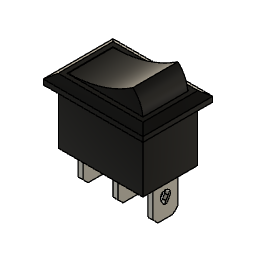
power_switch (Autodesk Fusion 360 design; units mm, degrees)
Autodesk Fusion 360 part; units mm, degrees
sketch "Main body" plane through (0, 0, 0) normal (0, 0, 1) x (1, 0, 0)
  line L0 (0, 0) -> (17, 0)
  line L1 (17, 0) -> (17, 11)
  line L2 (17, 11) -> (0, 11)
  line L3 (0, 11) -> (0, 0)
  dimension "d1" = 17
  dimension "d2" = 11
  constraint horizontal L0
  constraint vertical L1
  constraint horizontal L2
  constraint vertical L3
  constraint coincident L0.start L3.end
  measures "d1" distance of L0.start L0.end
  measures "d2" distance of L0.end L1.end
extrude "Extrude1" add sketch "Main body" along normal blind 11 makes body 1
sketch "Top Plate" plane through (0, 0, 11) normal (0, 0, 1) x (-1, 0, 0)
  line L0 (0, -11) -> (0, 0)
  line L1 (0, 0) -> (-17, 0)
  line L2 (-17, 0) -> (-17, -11)
  line L3 (-17, -11) -> (0, -11)
  line L4 (1.5, -12.5) -> (-18.5, -12.5)
  line L5 (-18.5, -12.5) -> (-18.5, 1.5)
  line L6 (-18.5, 1.5) -> (1.5, 1.5)
  line L7 (1.5, 1.5) -> (1.5, -12.5)
  dimension "d5" = 20
  dimension "d6" = 1.5
  dimension "d7" = 1.5
  dimension "d8" = 14
  dimension "d9" = 1.5
  dimension "d10" = 1.5
  constraint horizontal L4
  constraint vertical L5
  constraint horizontal L6
  constraint vertical L7
  measures "d5" distance of L5.end L6.end
  measures "d6" distance of L0 L7
  measures "d7" distance of L2 L5
  measures "d8" distance of L4.end L5.end
  measures "d9" distance of L3 L4
  measures "d10" distance of L1 L6
extrude "Extrude2" add sketch "Top Plate" along normal blind 2 contours L0 L1 L2 L3 | L4 L5 L6 L7 bodies 1
chamfer "Chamfer1" distance 1.5 distance2 1 1 edges at (8.5, -1.5, 13) measured on face at (11.8333, 7.8333, 13) on bodies 1
chamfer "Chamfer1" distance 1.5 distance2 1 3 edges at (18.5, 5.5, 13) (8.5, 12.5, 13) (-1.5, 5.5, 13) measured on face at (11.8333, 7.8333, 13) measured on face at (11.8333, 7.8333, 13) measured on face at (11.8333, 7.8333, 13) on bodies 1
sketch "Switch" plane through (0, 0, 13) normal (0, 0, 1) x (-1, 0, 0)
  line L0 (-17, -11) -> (0, -11)
  line L1 (0, -11) -> (0, 0)
  line L2 (0, 0) -> (-17, 0)
  line L3 (-17, 0) -> (-17, -11)
  line L4 (-1, -10) -> (-16, -10)
  line L5 (-16, -10) -> (-16, -1)
  line L6 (-16, -1) -> (-1, -1)
  line L7 (-1, -1) -> (-1, -10)
  line L8 (-0.9, -10.1) -> (-16.1, -10.1)
  line L9 (-16.1, -10.1) -> (-16.1, -0.9)
  line L10 (-16.1, -0.9) -> (-0.9, -0.9)
  line L11 (-0.9, -0.9) -> (-0.9, -10.1)
  line L12 (-16, -10) -> (-14, -10)
  line L13 (-14, -10) -> (-14, -1)
  line L14 (-14, -1) -> (-16, -1)
  line L15 (-16, -1) -> (-16, -10)
  dimension "d17" = 1
  dimension "d18" = 1
  dimension "d19" = 1
  dimension "d20" = 1
  dimension "d21" = 0.1
  dimension "d22" = 0.1
  dimension "d23" = 0.1
  dimension "d24" = 0.1
  dimension "d29" = 2
  constraint horizontal L4
  constraint vertical L5
  constraint horizontal L6
  constraint vertical L7
  constraint horizontal L8
  constraint vertical L9
  constraint horizontal L10
  constraint vertical L11
  constraint horizontal L12
  constraint vertical L13
  constraint horizontal L14
  constraint vertical L15
  constraint coincident L6 L13.end
  measures "d17" distance of L0 L4
  measures "d18" distance of L2 L6
  measures "d19" distance of L1 L7
  measures "d20" distance of L3 L5
  measures "d21" distance of L4 L8
  measures "d22" distance of L6 L10
  measures "d23" distance of L7 L11
  measures "d24" distance of L5 L9
  measures "d29" distance of L5 L13
extrude "Extrude3" cut sketch "Switch" against normal blind 1 contours L8 L9 L10 L11 bodies 1
extrude "Extrude4" add sketch "Switch" along normal blind 4 contours L4 L5 L6 L12 L13 L14 L15 bodies 1
fillet "Fillet1" radius 6.25 1 edges at (16, 5.5, 17) on bodies 1
fillet "Fillet2" radius 23.5 1 edges at (14, 5.5, 13) on bodies 1
sketch "Pins" plane through (0, 0, 0) normal (0, 0, -1) x (1, 0, 0)
  line L0 (0, 0) -> (0, -11)
  line L1 (0, -11) -> (17, -11)
  line L2 (17, -11) -> (17, 0)
  line L3 (17, 0) -> (0, 0)
  line L4 (1, -8) -> (2, -8)
  line L5 (2, -8) -> (2, -3)
  line L6 (2, -3) -> (1, -3)
  line L7 (1, -3) -> (1, -8)
  line L8 (8, -8) -> (9, -8)
  line L9 (9, -8) -> (9, -3)
  line L10 (9, -3) -> (8, -3)
  line L11 (8, -3) -> (8, -8)
  line L12 (15, -8) -> (16, -8)
  line L13 (16, -8) -> (16, -3)
  line L14 (16, -3) -> (15, -3)
  line L15 (15, -3) -> (15, -8)
  dimension "d34" = 5
  dimension "d37" = 1
  dimension "d38" = 1
  dimension "d39" = 1
  dimension "d40" = 1
  dimension "d41" = 1
  dimension "d42" = 6
  dimension "d43" = 6
  dimension "d44" = 3
  dimension "d45" = 3
  constraint horizontal L4
  constraint vertical L5
  constraint horizontal L6
  constraint vertical L7
  constraint horizontal L8
  constraint vertical L9
  constraint horizontal L10
  constraint vertical L11
  constraint horizontal L12
  constraint vertical L13
  constraint horizontal L14
  constraint vertical L15
  constraint collinear L6 L10
  constraint collinear L10 L14
  constraint collinear L4 L8
  constraint collinear L8 L12
  measures "d34" distance of L4.start L6.end
  measures "d37" distance of L8.start L8.end
  measures "d38" distance of L4.start L4.end
  measures "d39" distance of L12.start L12.end
  measures "d40" distance of L2 L13
  measures "d41" distance of L0 L7
  measures "d42" distance of L5 L11
  measures "d43" distance of L9 L15
  measures "d44" distance of L3 L6
  measures "d45" distance of L1 L4
extrude "Extrude5" add sketch "Pins" along normal blind 7 separate body contours L4 L5 L6 L7 | L8 L9 L10 L11 | L12 L13 L14 L15 makes body 2 at (1, 4.6667, -2.3333) makes body 3 at (8, 4.6667, -2.3333) makes body 4 at (15, 4.6667, -2.3333)
chamfer "Chamfer2" distance 1 angle 45 6 edges at (1.5, 3, -7) (1.5, 8, -7) (15.5, 3, -7) (15.5, 8, -7) (8.5, 3, -7) (8.5, 8, -7) on bodies 2 3 4
sketch "Right Pin Hole" plane through (16, 0, 0) normal (1, 0, 0) x (0, 1, 0)
  line L0 (7, -7) -> (8, -6)
  line L1 (8, -6) -> (8, 0)
  line L2 (8, 0) -> (3, 0)
  line L3 (3, 0) -> (3, -6)
  line L4 (3, -6) -> (4, -7)
  line L5 (4, -7) -> (7, -7)
  circle A0 through (6.4999, -3, -0.005) (5.0001, -2.134, 0.0218) (5, -3.866, 0.0089)
  circle A1 through (6.0012, -4, -0.0057) (5.2512, -3.567, 0.0077) (5.2512, -4.433, 0.0013)
  line L6 (5.9345, -4.2494, -0.0066) -> (6.3666, -3.4989, -0.0069)
  line L7 (5.0685, -4.2505, 0.0052) -> (4.6347, -3.5011, 0.0166)
  dimension "d49" = 2
  dimension "d50" = 4
  dimension "d51" = 2.5
  dimension "d52" = 1
sketch "Middle Pine Hole" plane through (9, 0, 0) normal (1, 0, 0) x (0, 1, 0)
  line L0 (7, -7) -> (8, -6)
  line L1 (8, -6) -> (8, 0)
  line L2 (8, 0) -> (3, 0)
  line L3 (3, 0) -> (3, -6)
  line L4 (3, -6) -> (4, -7)
  line L5 (4, -7) -> (7, -7)
  ellipse E0 centre (5.5, -3) end of major axis (5.9789, -2.1221) minor radius 0.9999
  ellipse E1 centre (5.5012, -4) end of major axis (5.7406, -3.561) minor radius 0.4999
  line L6 (5.9345, -4.2494) -> (6.3666, -3.4989)
  line L7 (5.0685, -4.2505) -> (4.6347, -3.5011)
sketch "Left Pin Hole" plane through (2, 0, 0) normal (1, 0, 0) x (0, 1, 0)
  line L0 (7, -7) -> (8, -6)
  line L1 (8, -6) -> (8, 0)
  line L2 (8, 0) -> (3, 0)
  line L3 (3, 0) -> (3, -6)
  line L4 (3, -6) -> (4, -7)
  line L5 (4, -7) -> (7, -7)
  ellipse E0 centre (5.5, -3) end of major axis (5.9789, -2.1221) minor radius 0.9999
  line L6 (5.0685, -4.2505) -> (4.6347, -3.5011)
  ellipse E1 centre (5.5012, -4) end of major axis (5.7406, -3.561) minor radius 0.4999
  line L7 (5.9345, -4.2494) -> (6.3666, -3.4989)
extrude "Extrude6" cut sketch "Left Pin Hole" against normal blind 1 contours E0 E1 | E0 L6 E1 | E0 E1 L7 | E0 E1 | E0 E1 bodies 2
extrude "Extrude7" cut sketch "Middle Pine Hole" against normal blind 1 contours E0 E1 | E0 E1 L7 | E0 E1 L6 | E0 E1 | E0 E1 bodies 3
extrude "Extrude8" cut sketch "Right Pin Hole" against normal blind 1 contours A0 A1 | A0 A1 L7 | A0 A1 L6 | A0 A1 | A0 A1 in plane through (16.1055, 0.0014, -0.0008) normal (0.99988, 0.01358, -0.007407) bodies 4
equation "d6 = ( ( 20 - 17 ) / 2 ) * 1 mm"
equation "d9 = ( ( 14 - 11 ) / 2 ) * 1 mm"
equation "d44 = ( ( 11 - 5 ) / 2 ) * 1 mm"
named bodies: "Main Body", "Left Pin", "Middle Pin", "Right Pin"
